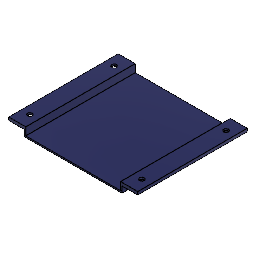
1-CBA bottom Cover V3 - part 3of3 v1 v4 (Autodesk Fusion 360 design; units mm, degrees)
Autodesk Fusion 360 part; units mm, degrees
sketch "extrusion" plane through (0, 0, 0) normal (0, 1, 0) x (1, 0, 0)
  line L0 (-82.5, -8) -> (-62.5, -8)
  line L1 (-62.5, -8) -> (-62.5, 0)
  line L2 (-62.5, 0) -> (62.5, 0)
  line L3 (62.5, 0) -> (62.5, -8)
  line L4 (62.5, -8) -> (82.5, -8)
  line L5 (-60.5, -12) -> (-60.5, -2)
  line L6 (-60.5, -2) -> (60.5, -2)
  line L7 (60.5, -2) -> (60.5, -12)
  line L8 (-82.5, -12) -> (-60.5, -12)
  line L9 (60.5, -12) -> (82.5, -12)
  line L10 (-82.5, -8) -> (-82.5, -12)
  line L11 (82.5, -8) -> (82.5, -12)
  dimension "d1" = 125
  dimension "d2" = 8
  dimension "d3" = 20
  dimension "d4" = 8
  dimension "d5" = 20
  constraint horizontal L0
  constraint perpendicular L0 L1
  constraint perpendicular L1 L2
  constraint perpendicular L2 L3
  constraint perpendicular L1 L4
  constraint midpoint origin L2
  constraint parallel L1 L5
  constraint parallel L2 L6
  constraint parallel L3 L7
  constraint parallel L4 L9
  constraint parallel L0 L8
  constraint perpendicular L8 L10
  constraint perpendicular L9 L11
  measures "d1" distance of L1.end L2.end
  measures "d2" distance of L0.end L1.end
  measures "d3" distance of L0.start L0.end
  measures "d4" distance of L2.end L3.end
  measures "d5" distance of L3.end L4.end
extrude "Extrude1" add sketch "extrusion" along normal mid plane 140
sketch "top holes" plane through (0, 0, 12) normal (0, 0, 1) x (-1, 0, 0)
  circle A0 centre (71.5, -53.75) radius 3
  line L0 (82.5, -70) -> (60.5, -70)
  point P0 (71.5, -70)
  dimension "d11" = 6
  dimension "d12" = 16.25
  constraint midpoint L0 P0
  constraint vertical A0.centre P0
  measures "d11" diameter of A0
  measures "d12" distance of A0.centre L0
extrude "Extrude2" cut sketch "top holes" against normal blind 4
mirror "Mirror1" about plane through (0, 0, 0) normal (1, 0, 0) of "Extrude2"
mirror "Mirror2" about plane through (0, 0, 0) normal (0, 1, 0) of "Extrude2", "Mirror1"
sketch "Sketch5" plane through (0, 0, 8) normal (0, 0, -1) x (1, 0, 0)
  circle A0 centre (71.5, 53.75) radius 3
  circle A1 centre (71.5, -53.75) radius 3
  line L0 (62.5, 70) -> (62.5, -70)
  line L1 (62.5, -70) -> (82.5, -70)
  line L2 (82.5, -70) -> (82.5, 70)
  line L3 (82.5, 70) -> (62.5, 70)
  circle A2 centre (71.5, 53.75) radius 5
  dimension "d35" = 10
  constraint concentric A0 A2
  measures "d35" diameter of A2
extrude "Extrude6" cut sketch "Sketch5" against normal blind 2 contours A2
sketch "Sketch6" plane through (0, 0, 8) normal (0, 0, -1) x (1, 0, 0)
  circle A0 centre (71.5, 53.75) radius 5
  circle A1 centre (71.5, -53.75) radius 3
  line L0 (62.5, 70) -> (62.5, -70)
  line L1 (62.5, -70) -> (82.5, -70)
  line L2 (82.5, -70) -> (82.5, 70)
  line L3 (82.5, 70) -> (62.5, 70)
  circle A2 centre (71.5, -53.75) radius 5
  dimension "d38" = 10
  constraint concentric A1 A2
  measures "d38" diameter of A2
extrude "Extrude7" cut sketch "Sketch6" against normal blind 2 contours A2
sketch "Sketch7" plane through (0, 0, 8) normal (0, 0, -1) x (1, 0, 0)
  circle A0 centre (-71.5, 53.75) radius 3
  circle A1 centre (-71.5, -53.75) radius 3
  line L0 (-82.5, 70) -> (-82.5, -70)
  line L1 (-82.5, -70) -> (-62.5, -70)
  line L2 (-62.5, -70) -> (-62.5, 70)
  line L3 (-62.5, 70) -> (-82.5, 70)
  circle A2 centre (-71.5, 53.75) radius 5
  dimension "d41" = 10
  constraint concentric A0 A2
  measures "d41" diameter of A2
extrude "Extrude8" cut sketch "Sketch7" against normal blind 2 contours A2
sketch "Sketch8" plane through (0, 0, 8) normal (0, 0, -1) x (1, 0, 0)
  circle A0 centre (-71.5, 53.75) radius 5
  circle A1 centre (-71.5, -53.75) radius 3
  line L0 (-82.5, 70) -> (-82.5, -70)
  line L1 (-82.5, -70) -> (-62.5, -70)
  line L2 (-62.5, -70) -> (-62.5, 70)
  line L3 (-62.5, 70) -> (-82.5, 70)
  circle A2 centre (-71.5, -53.75) radius 5
  dimension "d44" = 10
  constraint concentric A1 A2
  measures "d44" diameter of A2
extrude "Extrude9" cut sketch "Sketch8" against normal blind 2 contours A2
